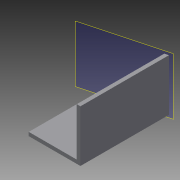
# Autodesk Inventor part: ring support right
Saved by Autodesk Inventor 2014 SP1 (Build 180222100, 222)
## iProperties
Created: 2015-02-06
Part Number: ring support right
Material: Generic
Document SubType Name: Modeling
Designer: degan
Density: 1 g/cm^3
Appearance: Default
Author: degan
Autodesk Inventor part; units mm, degrees
ref_plane "YZ Plane" through (0, 0, 0) normal (1, 0, 0) x (0, 1, 0)
ref_plane "XZ Plane" through (0, 0, 0) normal (0, 1, 0) x (-1, 0, 0)
ref_plane "XY Plane" through (0, 0, 0) normal (0, 0, 1) x (1, 0, 0)
sketch "Sketch1" plane through (0, 0, 0) normal (0, 0, 1) x (1, 0, 0)
  line L0 (0, 0) -> (0, 44.45)
  line L1 (0, 0) -> (-44.45, 0)
  line L2 (-3.175, 44.45) -> (-3.175, 3.175)
  line L3 (-3.175, 3.175) -> (-44.45, 3.175)
  line L4 (-3.175, 44.45) -> (0, 44.45)
  line L5 (-44.45, 3.175) -> (-44.45, 0)
  dimension "d0" = 44.45
  dimension "d1" = 44.45
  dimension "d2" = 3.175
  constraints: 12 end point, 3 perpendicular, 1 parallel, 1 vertical, 1 other
  measures "d0" distance of L0.start L0.end
  measures "d1" distance of L0.start L1.end
  measures "d2" distance between parallel lines of L0 L2
extrude "Extrusion1" add sketch "Sketch1" along normal blind 76.2
ref_plane "Work Plane1" through (0, 0, 0) normal (-0.2588, 0, -0.9659) x (0, 1, 0)
split "Split1" plane through (0, 0, 0) removes the side toward (-0.2588, 0, -0.9659)
body "Solid1"
